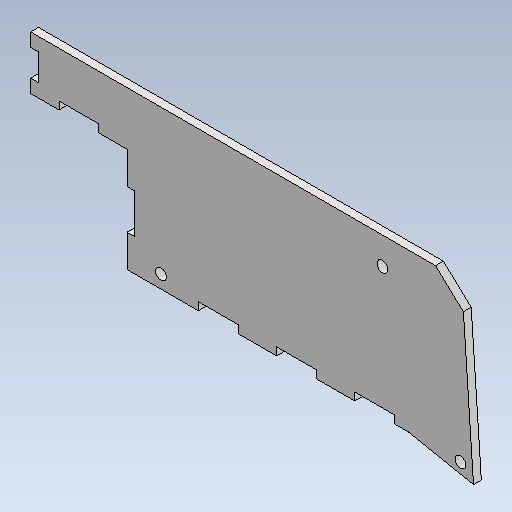
# Autodesk Inventor part: bed_acrylic_side
Saved by Autodesk Inventor 2025 (Build 290162000, 162)
## iProperties
Created: 2025-08-24
Part Number: bed_acrylic_side
Material: Generic
Document SubType Name: Modeling
Designer: HP
Density: 1 g/cm^3
Appearance: Default
Author: HP
Autodesk Inventor part; units mm, degrees
ref_plane "YZ Plane" through (0, 0, 0) normal (1, 0, 0) x (0, 1, 0)
ref_plane "XZ Plane" through (0, 0, 0) normal (0, 1, 0) x (-1, 0, 0)
ref_plane "XY Plane" through (0, 0, 0) normal (0, 0, 1) x (1, 0, 0)
sketch "Sketch1" plane through (0, 0, 0) normal (0, 0, 1) x (1, 0, 0)
  line L0 (-66.5, -32.75) -> (66.5, -32.75)
  line L1 (66.5, -32.75) -> (66.5, 32.75)
  line L2 (66.5, 32.75) -> (-66.5, 32.75)
  line L3 (-66.5, 32.75) -> (-66.5, -32.75)
  line L4 (-66.5, -32.75) -> (66.5, 32.75) construction
  line L5 (66.5, -32.75) -> (-66.5, 32.75) construction
  line L6 (-103.5, 32.75) -> (-66.5, 32.75)
  line L7 (-66.5, 32.75) -> (-66.5, 12.25)
  line L8 (-66.5, 12.25) -> (-103.5, 12.25)
  line L9 (-103.5, 12.25) -> (-103.5, 32.75)
  line L10 (-103.5, 32.75) -> (-66.5, 12.25) construction
  line L11 (-66.5, 32.75) -> (-103.5, 12.25) construction
  line L12 (66.5, -32.75) -> (61.9198, 32.75)
  circle A0 centre (-53.5, -22.75) radius 2.1
  circle A1 centre (31.5, 22.25) radius 2.1
  line L13 (-66.5, -27.75) -> (41.5, -27.75)
  line L14 (41.5, -27.75) -> (66.5, -32.75)
  circle A2 centre (61.5, -27.75) radius 2.1
  point P0 (0, 0)
  point P1 (-85, 22.5)
  dimension "d0" = 65.5
  dimension "d1" = 133
  dimension "d3" = 37
  dimension "d4" = 4.2
  dimension "d5" = 13
  dimension "d7" = 98
  dimension "d8" = 108
  dimension "d9" = 5
  dimension "d10" = 5
  dimension "d11" = 50
  dimension "d12" = 4.2
  dimension "d13" = 4.2
  dimension "d15" = 5
  dimension "d16" = 4
  dimension "d36" = 40
  constraints: 30 end point, 4 midpoint, 4 parallel, 3 centre point, 3 horizontal, 3 point on line, 2 collinear, 2 perpendicular
  measures "d0" distance between parallel lines of L0 L2
  measures "d1" distance between parallel lines of L1 L3
  measures "d3" distance between parallel lines of L3 L9
  measures "d4" diameter of A0
  measures "d5" distance from line of L3 A0.centre
  measures "d7" distance from line of L3 A1.centre
  measures "d8" distance of L13.start L13.end
  measures "d9" distance between parallel lines of L0 L13
  measures "d10" distance from line of L13 A0.centre
  measures "d11" distance from line of L13 A1.centre
  measures "d12" diameter of A1
  measures "d13" diameter of A2
  measures "d15" distance from line of L1 A2.centre
  measures "d16" angle of L1 L12
  measures "d36" distance between parallel lines of L8 L13
extrude "Extrusion1" add sketch "Sketch1" along normal blind 3 contours L14 L13 L3 L2 L12 | L8 L9 L6 L3
sketch "Sketch2" plane through (0, 0, 3) normal (0, 0, 1) x (1, 0, 0)
  line L0 (66.5, -32.75) -> (61.9198, 32.75) construction
  line L1 (61.9198, 32.75) -> (-103.5, 32.75) construction
  line L2 (-103.5, 32.75) -> (-103.5, 12.25) construction
  line L3 (-103.5, 12.25) -> (-66.5, 12.25) construction
  line L4 (-66.5, 12.25) -> (-66.5, -27.75) construction
  line L5 (-66.5, -27.75) -> (41.5, -27.75) construction
  line L6 (41.5, -27.75) -> (66.5, -32.75) construction
  circle A0 centre (-53.5, -22.75) radius 2.1 construction
  circle A1 centre (31.5, 22.25) radius 2.1 construction
  circle A2 centre (61.5, -27.75) radius 2.1 construction
  line L7 (-103.5, 27.6) -> (-100.5, 27.6)
  line L8 (-100.5, 27.6) -> (-100.5, 17.4)
  line L9 (-100.5, 17.4) -> (-103.5, 17.4)
  line L10 (-103.5, 17.4) -> (-103.5, 27.6)
  line L11 (-103.5, 27.6) -> (-100.5, 17.4) construction
  line L12 (-100.5, 27.6) -> (-103.5, 17.4) construction
  line L13 (-92.6, 12.25) -> (-77.4, 12.25)
  line L14 (-77.4, 12.25) -> (-77.4, 15.25)
  line L15 (-77.4, 15.25) -> (-92.6, 15.25)
  line L16 (-92.6, 15.25) -> (-92.6, 12.25)
  line L17 (-92.6, 12.25) -> (-77.4, 15.25) construction
  line L18 (-77.4, 12.25) -> (-92.6, 15.25) construction
  line L19 (-103.5, 12.25) -> (-66.5, 12.25) projected
  line L20 (-66.5, -15.35) -> (-63.5, -15.35)
  line L21 (-63.5, -15.35) -> (-63.5, -0.15)
  line L22 (-63.5, -0.15) -> (-66.5, -0.15)
  line L23 (-66.5, -0.15) -> (-66.5, -15.35)
  line L24 (-66.5, -15.35) -> (-63.5, -0.15) construction
  line L25 (-63.5, -15.35) -> (-66.5, -0.15) construction
  line L26 (-66.5, 12.25) -> (-66.5, -27.75) projected
  line L27 (-39.1, -27.75) -> (-23.9, -27.75)
  line L28 (-23.9, -27.75) -> (-23.9, -24.75)
  line L29 (-23.9, -24.75) -> (-39.1, -24.75)
  line L30 (-39.1, -24.75) -> (-39.1, -27.75)
  line L31 (-39.1, -27.75) -> (-23.9, -24.75) construction
  line L32 (-23.9, -27.75) -> (-39.1, -24.75) construction
  line L33 (-66.5, -27.75) -> (41.5, -27.75) projected
  line L34 (-9.1, -27.75) -> (6.1, -27.75)
  line L35 (6.1, -27.75) -> (6.1, -24.75)
  line L36 (6.1, -24.75) -> (-9.1, -24.75)
  line L37 (-9.1, -24.75) -> (-9.1, -27.75)
  line L38 (-9.1, -27.75) -> (6.1, -24.75) construction
  line L39 (6.1, -27.75) -> (-9.1, -24.75) construction
  line L40 (20.9, -27.75) -> (36.1, -27.75)
  line L41 (36.1, -27.75) -> (36.1, -24.75)
  line L42 (36.1, -24.75) -> (20.9, -24.75)
  line L43 (20.9, -24.75) -> (20.9, -27.75)
  line L44 (20.9, -27.75) -> (36.1, -24.75) construction
  line L45 (36.1, -27.75) -> (20.9, -24.75) construction
  point P0 (0, 0)
  point P1 (-102, 22.5)
  point P2 (-103.5, 22.5)
  point P3 (-85, 13.75)
  point P4 (-85, 12.25)
  point P5 (-65, -7.75)
  point P6 (-66.5, -7.75)
  point P7 (-31.5, -26.25)
  point P8 (-1.5, -26.25)
  point P9 (28.5, -26.25)
  point P10 (20.9, -27.75)
  point P11 (36.1, -27.75)
  point P12 (-9.1, -27.75)
  point P13 (6.1, -27.75)
  dimension "d19" = 3
  dimension "d20" = 10.2
  dimension "d21" = 3
  dimension "d22" = 15.2
  dimension "d23" = 3
  dimension "d24" = 15.2
  dimension "d25" = 3
  dimension "d26" = 15.2
  dimension "d27" = 3
  dimension "d28" = 15.2
  dimension "d30" = 35
  dimension "d31" = 3
  dimension "d33" = 15.2
  dimension "d37" = 30
  dimension "d38" = 30
  constraints: 72 end point, 15 midpoint, 12 parallel, 6 collinear, 6 horizontal, 6 perpendicular, 2 horizontal alignment, 1 vertical alignment
  measures "d19" distance of L8.end L9.end
  measures "d20" distance between parallel lines of L9 L7
  measures "d21" distance between parallel lines of L13 L15
  measures "d22" distance between parallel lines of L14 L16
  measures "d23" distance between parallel lines of L21 L23
  measures "d24" distance between parallel lines of L20 L22
  measures "d25" distance between parallel lines of L27 L29
  measures "d26" distance between parallel lines of L28 L30
  measures "d27" distance between parallel lines of L34 L36
  measures "d28" distance between parallel lines of L35 L37
  measures "d30" distance from line of L4 point (-31.5, -26.25)
  measures "d31" distance between parallel lines of L40 L42
  measures "d33" distance between parallel lines of L41 L43
  measures "d37" distance of point (-1.5, -26.25) point (-31.5, -26.25)
  measures "d38" distance of point (28.5, -26.25) point (-1.5, -26.25)
extrude "Extrusion2" cut sketch "Sketch2" against normal through all
chamfer "Chamfer1" distance 10 angle 45 1 edges at (61.9198, 32.75, 1.5)
equation "\"d12\" = d4"
equation "\"d13\" = d12"
equation "\"d21\" = d19"
equation "\"d23\" = d21"
equation "\"d25\" = d23"
equation "\"d27\" = d25"
equation "\"d28\" = d26"
equation "\"d31\" = d27"
equation "\"d33\" = d28"
equation "\"d38\" = d37"
body "Solid1"
